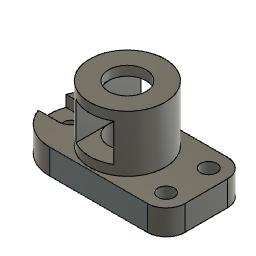
drawing_9 v1 (Autodesk Fusion 360 design; units mm, degrees)
Autodesk Fusion 360 part; units mm, degrees
note: some values were not read from the file. Set by a fixed rule: which sketch regions a step uses.
sketch "Sketch3" plane through (0, 0, 0) normal (0, 1, 0) x (1, 0, 0)
  line L0 (42, -10) -> (120, -10)
  line L1 (135, -25) -> (135, -59)
  line L2 (120, -74) -> (42, -74)
  line L3 (10, -42) -> (10, -42)
  arc A0 (42, -10) -> (10, -42) centre (42, -42) ccw
  arc A1 (10, -42) -> (42, -74) centre (42, -42) ccw
  arc A2 (135, -25) -> (120, -10) centre (120, -25) ccw
  arc A3 (120, -74) -> (135, -59) centre (120, -59) ccw
  circle A4 centre (120, -59) radius 6.5
  circle A5 centre (120, -25) radius 6.5
  point P0 (10, -10)
  point P1 (135, -10)
  point P2 (10, -74)
  dimension "d17" = 125
  dimension "d18" = 64
  dimension "d19" = 32
  dimension "d20" = 32
  dimension "d21" = 15
  dimension "d22" = 15
  dimension "d23" = 13
  dimension "d24" = 13
  constraint horizontal L0
  constraint vertical L1
  constraint horizontal L2
  constraint coincident P0 L0
  constraint tangent L0 A0
  constraint coincident P2 L2
  constraint coincident P2 L3
  constraint tangent L2 A1
  constraint coincident P1 L0
  constraint coincident P1 L1
  constraint tangent L0 A2
  constraint tangent L1 A2
  constraint tangent L1 A3
  constraint tangent L2 A3
  measures "d17" distance of P0 P1
  measures "d18" distance of P0 P2
  measures "d19" radius of A0
  measures "d20" radius of A1
  measures "d21" radius of A2
  measures "d22" radius of A3
  measures "d23" diameter of A4
  measures "d24" diameter of A5
extrude "Extrude3" add sketch "Sketch3" along normal blind 20
sketch "Sketch4" plane through (0, 20, 0) normal (0, 1, 0) x (-1, 0, 0)
  circle A0 centre (-120, 59) radius 6.5
  circle A1 centre (-120, 25) radius 6.5
  arc A2 (-42, 10) -> (-42, 74) centre (-42, 42) ccw
  line L0 (-42, 74) -> (-120, 74)
  arc A3 (-120, 74) -> (-135, 59) centre (-120, 59) ccw
  line L1 (-135, 59) -> (-135, 25)
  arc A4 (-135, 25) -> (-120, 10) centre (-120, 25) ccw
  line L2 (-120, 10) -> (-42, 10)
  line L3 (-120, 59) -> (-72, 59)
  line L4 (-120, 25) -> (-72, 25)
  line L5 (-72, 59) -> (-72, 25)
  line L6 (-72, 59) -> (-72, 42)
  circle A5 centre (-72, 42) radius 30
  dimension "d27" = 48
  dimension "d28" = 48
  dimension "d29" = 60
  constraint coincident A0.centre A3.centre
  constraint horizontal L3
  constraint coincident A1.centre A4.centre
  constraint horizontal L4
  constraint midpoint L5 L6.end
  constraint coincident L6.end A5.centre
  measures "d27" distance of A0.centre L3.end
  measures "d28" distance of A1.centre L4.end
  measures "d29" diameter of A5
extrude "Extrude4" add sketch "Sketch4" along normal blind 45 contours L3 L4 L5 L6 A5 | L3 L4 L5 L6 A5
hole "Hole1" at (72, 65, 42) direction (0, -1, 0) diameter 30 depth 90 tip angle 118
sketch "Sketch5" plane through (0, 0, 74) normal (0, 0, 1) x (1, 0, 0)
  line L0 (42, 0) -> (120, 0)
  line L1 (120, 0) -> (120, 20)
  line L2 (120, 20) -> (42, 20)
  line L3 (42, 20) -> (42, 0)
sketch "Sketch6" plane through (0, 0, 0) normal (0, 0, 1) x (1, 0, 0)
  line L0 (42, 65) -> (72, 65)
  line L1 (42, 65) -> (42, 57.5)
  line L2 (42, 57.5) -> (57, 57.5)
  line L3 (57, 57.5) -> (87, 57.5)
  line L4 (87, 57.5) -> (87, 27.5)
  line L5 (87, 27.5) -> (57, 27.5)
  line L6 (57, 27.5) -> (57, 57.5)
  dimension "d35" = 30
  dimension "d36" = 7.5
  dimension "d37" = 30
  dimension "d38" = 30
  constraint horizontal L0
  constraint perpendicular L0 L1
  constraint perpendicular L1 L2
  constraint horizontal L3
  constraint vertical L4
  constraint horizontal L5
  constraint vertical L6
  measures "d35" distance of L0.start L0.end
  measures "d36" distance of L0.start L1.end
  measures "d37" distance of L2.end L3.end
  measures "d38" distance of L2.end L5.end
extrude "Extrude5" cut sketch "Sketch6" along normal blind 200
sketch "Sketch7" plane through (0, 0, 0) normal (0, 1, 0) x (1, 0, 0)
sketch "Sketch8" plane through (0, 20, 0) normal (0, 1, 0) x (-1, 0, 0)
  circle A0 centre (-72, 42) radius 30
  circle A1 centre (-120, 59) radius 6.5
  circle A2 centre (-120, 25) radius 6.5
  arc A3 (-42, 10) -> (-42, 74) centre (-42, 42) ccw
  line L0 (-42, 74) -> (-120, 74)
  arc A4 (-120, 74) -> (-135, 59) centre (-120, 59) ccw
  line L1 (-135, 59) -> (-135, 25)
  arc A5 (-135, 25) -> (-120, 10) centre (-120, 25) ccw
  line L2 (-120, 10) -> (-42, 10)
  line L3 (-72, 42) -> (-27, 42)
  circle A6 centre (-27, 42) radius 6.5
  dimension "d41" = 45
  dimension "d42" = 13
  constraint coincident A0.centre L3.start
  constraint horizontal L3
  constraint coincident L3.end A6.centre
  measures "d41" distance of A0.centre L3.end
  measures "d42" diameter of A6
extrude "Extrude6" cut sketch "Sketch8" against normal blind 9 contours A6
sketch "Sketch9" plane through (0, 20, 0) normal (0, 1, 0) x (-1, 0, 0)
  circle A0 centre (-27, 42) radius 6.5
  circle A1 centre (-72, 42) radius 30
  circle A2 centre (-120, 59) radius 6.5
  circle A3 centre (-120, 25) radius 6.5
  arc A4 (-42, 10) -> (-42, 74) centre (-42, 42) ccw
  line L0 (-42, 74) -> (-120, 74)
  arc A5 (-120, 74) -> (-135, 59) centre (-120, 59) ccw
  line L1 (-135, 59) -> (-135, 25)
  arc A6 (-135, 25) -> (-120, 10) centre (-120, 25) ccw
  line L2 (-120, 10) -> (-42, 10)
  line L3 (-27, 42) -> (-27, 31)
  line L4 (-27, 31) -> (-6.9654, 31)
  line L5 (-6.9654, 31) -> (-6.9654, 50)
  line L6 (-6.9654, 50) -> (-6.9654, 31)
  line L7 (-27, 42) -> (-27, 53)
  line L8 (-27, 53) -> (-28, 53)
  line L9 (-38, 43) -> (-38, 41)
  line L10 (-38, 31) -> (-27, 31)
  line L11 (-27, 31) -> (-27, 53)
  line L12 (-28, 31) -> (-6, 31)
  line L13 (-6, 31) -> (-6, 53)
  line L14 (-6, 53) -> (-38, 53)
  line L15 (-38, 53) -> (-38, 31)
  arc A7 (-38, 41) -> (-28, 31) centre (-28, 41) ccw
  arc A8 (-28, 53) -> (-38, 43) centre (-28, 43) ccw
  point P0 (-38, 53)
  dimension "d45" = 11
  dimension "d46" = 11
  dimension "d47" = 11
  dimension "d48" = 22
  dimension "d49" = 32
  dimension "d50" = 22
  dimension "d51" = 10
  dimension "d52" = 10
  constraint coincident A0.centre L3.start
  constraint vertical L3
  constraint perpendicular L3 L4
  constraint perpendicular L4 L5
  constraint parallel L3 L7
  constraint horizontal L8
  constraint vertical L9
  constraint horizontal L10
  constraint vertical L11
  constraint horizontal L12
  constraint vertical L13
  constraint horizontal L14
  constraint vertical L15
  constraint coincident L10.start L12
  constraint coincident L10.start L9
  constraint tangent L12 A7
  constraint tangent L9 A7
  constraint coincident P0 L8
  constraint coincident P0 L9
  constraint tangent L8 A8
  constraint tangent L9 A8
  measures "d45" distance of A0.centre L3.end
  measures "d46" distance of A0.centre L7.end
  measures "d47" distance of L7.end P0
  measures "d48" distance of L7.end L3.end
  measures "d49" distance of L10.start L12.end
  measures "d50" distance of L10.start P0
  measures "d51" radius of A7
  measures "d52" radius of A8
extrude "Extrude7" cut sketch "Sketch9" against normal blind 9 contours A0 A4 L3 L4 L7 L11 L12 L14 | A0 L3 L7 L8 L9 L10 L11 L12 L14 L15 A7 A8
hole "Hole2" at (27.171, 11, 42.0282) direction (0, -1, 0) diameter 12 depth 13 tip angle 118
